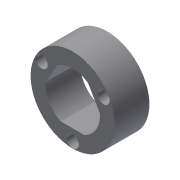
# Autodesk Inventor part: cellSTORM_magnetic_RMS_adapter
Saved by Autodesk Inventor 2019 (Build 230136000, 136)
## iProperties
Created: 2020-02-12
Part Number: cellSTORM_magnetic_RMS_adapter
Material: Generic
Document SubType Name: Modeling
Designer: diederichbenedict
Density: 1 g/cm^3
Appearance: Default
Author: diederichbenedict
Autodesk Inventor part; units mm, degrees
ref_plane "YZ Plane" through (0, 0, 0) normal (1, 0, 0) x (0, 1, 0)
ref_plane "XZ Plane" through (0, 0, 0) normal (0, 1, 0) x (-1, 0, 0)
ref_plane "XY Plane" through (0, 0, 0) normal (0, 0, 1) x (1, 0, 0)
sketch "Sketch1" plane through (0, 0, 0) normal (0, 0, 1) x (1, 0, 0)
  circle A0 centre (0, 0) radius 17
  line L0 (4.7948, -9.9) -> (-4.7948, -9.9)
  line L1 (-23.8, 0) -> (23.8, 0) projected
  line L2 (6.1763, 9.1024) -> (10.971, 0.7976)
  line L3 (-10.971, 0.7976) -> (-6.1763, 9.1024)
  arc A1 (4.7948, -9.9) -> (10.971, 0.7976) centre (0, 0) ccw
  arc A2 (6.1763, 9.1024) -> (-6.1763, 9.1024) centre (0, 0) ccw
  arc A3 (-10.971, 0.7976) -> (-4.7948, -9.9) centre (0, 0) ccw
  dimension "d1" = 34
  dimension "d2" = 9.9
  dimension "d5" = 360
  dimension "d18" = 11
  constraints: 6 end point, 6 point on circle, 4 centre point, 2 coincident, 1 parallel, 10 other
  measures "d1" diameter of A0
  measures "d2" distance from line of L0 point (0, 0)
  measures "d18" radius of A1
extrude "Extrusion1" add sketch "Sketch1" along normal blind 4 contours L1 A1 L2 A2 L3 A3 A0 | A0 L1 A3 L0 A1
sketch "Sketch3" plane through (0, 0, 4) normal (0, 0, 1) x (1, 0, 0)
  arc A0 (-12.5839, 8.6144) -> (-13.7522, 6.5908) centre (-12.5, 7.2169) ccw projected
  arc A1 (12.9288, 8.5496) -> (13.8686, 6.9219) centre (12.5, 7.2169) ccw projected
  arc A2 (0.9397, -15.4715) -> (-0.9397, -15.4715) centre (0, -14.4338) ccw projected
  point P0 (0, 0)
hole "Hole1" at (12.5, 7.2169, 4) at (0, -14.4338, 4) at (-12.5, 7.2169, 4) direction (0, 0, -1) diameter 4.9 depth 3 tip angle 118
sketch "Sketch4" plane through (0, 0, 0) normal (0, 0, -1) x (-1, 0, 0)
  circle A0 centre (0, -14.4338) radius 0.7857 projected
  circle A1 centre (-12.5, 7.2169) radius 0.7857 projected
  circle A2 centre (12.5, 7.2169) radius 0.7857 projected
  arc A3 (4.7948, -9.9) -> (10.971, 0.7976) centre (0, 0) ccw projected
  line L0 (4.7948, -9.9) -> (-4.7948, -9.9) projected
  arc A4 (-10.971, 0.7976) -> (-4.7948, -9.9) centre (0, 0) ccw projected
  line L1 (-10.971, 0.7976) -> (-6.1763, 9.1024) projected
  arc A5 (6.1763, 9.1024) -> (-6.1763, 9.1024) centre (0, 0) ccw projected
  line L2 (6.1763, 9.1024) -> (10.971, 0.7976) projected
  circle A6 centre (0, 0) radius 17 projected
extrude "Extrusion2" add sketch "Sketch4" along normal blind 10 contours A0 | A1 | A2 | A6
body "Solid1"
